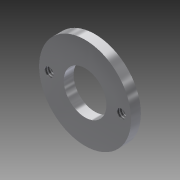
# Autodesk Inventor part: Pneumatic Connector Cap
Saved by Autodesk Inventor 2013 (Build 170138000, 138)
## iProperties
Created: 2013-08-25
Part Number: Pneumatic Connector Cap
Material: Generic
Document SubType Name: Modeling
Designer: grtstudent
Density: 1 g/cm^3
Author: grtstudent
Autodesk Inventor part; units mm, degrees
ref_plane "YZ Plane" through (0, 0, 0) normal (1, 0, 0) x (0, 1, 0)
ref_plane "XZ Plane" through (0, 0, 0) normal (0, 1, 0) x (-1, 0, 0)
ref_plane "XY Plane" through (0, 0, 0) normal (0, 0, 1) x (1, 0, 0)
sketch "Sketch1" plane through (0, 0, 0) normal (0, 0, 1) x (1, 0, 0)
  circle A0 centre (0, 0) radius 11.1125
  circle A1 centre (0, 0) radius 5.1594
  circle A2 centre (0, 0) radius 6.35 construction
  circle A3 centre (0, 0) radius 8.7313 construction
  line L0 (-8.7313, 0) -> (8.7313, 0) construction
  dimension "d0" = 22.225
  dimension "d2" = 10.3187
  dimension "d6" = 12.7
  dimension "d7" = 2.3813
  dimension "d8" = 2.3813
  constraints: 4 centre point, 4 coincident, 2 end point, 2 point on circle, 1 horizontal, 1 midpoint
  measures "d0" diameter of A0
  measures "d2" diameter of A1
  measures "d6" diameter of A2
  measures "d7" radial gap between concentric circles of A2 A3
  measures "d8" radial gap between concentric circles of A3 A0
extrude "Extrusion1" add sketch "Sketch1" along normal blind 2.3813
hole "Hole1" at (-8.7313, 0, 0) at (8.7313, 0, 0) direction (0, 0, 1) diameter 2.159 end through all
equation "\"d7\" = d8"
body "Solid1"
